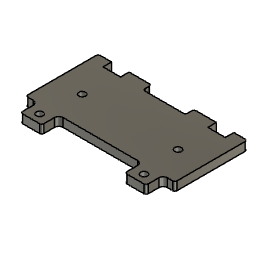
headcamera_plate_1 (Autodesk Fusion 360 design; units mm, degrees)
Autodesk Fusion 360 part; units mm, degrees
note: some values were not read from the file. Set by a fixed rule: the direction of a hole.
sketch "スケッチ1" plane through (0, 0, 0) normal (0, 0, 1) x (1, 0, 0)
  line L0 (-20.5, 20) -> (20.5, 20)
  line L1 (20.5, 20) -> (20.5, 16)
  line L2 (20.5, 16) -> (28.7, 16)
  line L3 (28.7, 16) -> (28.7, 20)
  line L4 (28.7, 20) -> (35, 20)
  line L5 (35, 20) -> (35, -14)
  line L6 (35, -14) -> (29.5, -14)
  line L7 (29.5, -14) -> (29.5, -22)
  line L8 (29.5, -22) -> (19.5, -22)
  line L9 (19.5, -22) -> (19.5, -14)
  line L10 (19.5, -14) -> (-19.5, -14)
  line L11 (-19.5, -14) -> (-19.5, -22)
  line L12 (-19.5, -22) -> (-29.5, -22)
  line L13 (-29.5, -22) -> (-29.5, -14)
  line L14 (-29.5, -14) -> (-35, -14)
  line L15 (-35, -14) -> (-35, 20)
  line L16 (-35, 20) -> (-28.7, 20)
  line L17 (-28.7, 20) -> (-28.7, 16)
  line L18 (-28.7, 16) -> (-20.5, 16)
  line L19 (-20.5, 16) -> (-20.5, 20)
  line L20 (-22.5, 0) -> (22.5, 0)
  line L21 (-24.5, -22) -> (-24.5, -18)
  line L22 (24.5, -22) -> (24.5, -18)
  line L23 (-10, 16) -> (10, 16)
  line L24 (10, 16) -> (10, 20)
  line L25 (10, 20) -> (-10, 20)
  line L26 (-10, 20) -> (-10, 16)
  point P0 (0, 20)
  point P1 (0, -14)
  dimension "d1" = 16
  dimension "d2" = 4
  dimension "d4" = 14
  dimension "d5" = 8
  dimension "d6" = 41
  dimension "d7" = 8.2
  dimension "d8" = 8.2
  dimension "d9" = 70
  dimension "d10" = 45
  dimension "d16" = 39
  dimension "d17" = 10
  dimension "d18" = 10
  dimension "d19" = 4
  dimension "d24" = 20
  dimension "d25" = 4
  constraint horizontal L0
  constraint perpendicular L0 L1
  constraint perpendicular L1 L2
  constraint perpendicular L2 L3
  constraint perpendicular L3 L4
  constraint perpendicular L4 L5
  constraint perpendicular L5 L6
  constraint perpendicular L4 L7
  constraint perpendicular L5 L8
  constraint perpendicular L8 L9
  constraint perpendicular L9 L10
  constraint perpendicular L8 L11
  constraint perpendicular L11 L12
  constraint perpendicular L8 L13
  constraint perpendicular L13 L14
  constraint perpendicular L14 L15
  constraint perpendicular L15 L16
  constraint perpendicular L16 L17
  constraint perpendicular L15 L18
  constraint perpendicular L0 L19
  constraint coincident L0.start L19.end
  constraint midpoint L0 P0
  constraint midpoint L10 P1
  constraint vertical origin P1
  constraint vertical origin P0
  constraint collinear L2 L18
  constraint collinear L0 L16
  constraint collinear L0 L4
  constraint collinear L6 L10
  constraint collinear L10 L14
  constraint collinear L8 L12
  constraint equal L4 L16
  constraint horizontal L20
  constraint midpoint origin L20
  constraint midpoint L12 L21.start
  constraint perpendicular L12 L21
  constraint midpoint L8 L22.start
  constraint perpendicular L8 L22
  constraint equal L21 L22
  constraint horizontal L23
  constraint vertical L24
  constraint horizontal L25
  constraint vertical L26
  constraint midpoint P0 L25
  measures "d1" distance of origin L2
  measures "d2" distance of L2.end L3.end
  measures "d4" distance of origin L6
  measures "d5" distance of L6 L8
  measures "d6" distance of L0.start L0.end
  measures "d7" distance of L1.end L2.end
  measures "d8" distance of L17.end L18.end
  measures "d9" distance of L5 L15
  measures "d10" distance of L20.start L20.end
  measures "d16" distance of L9.end L10.end
  measures "d17" distance of L11.end L12.end
  measures "d18" distance of L7 L9
  measures "d19" distance of L21.start L21.end
  measures "d24" distance of L24 L26
  measures "d25" distance of L23.end L24.end
extrude "押し出し1" add sketch "スケッチ1" along normal blind 4 contours L0 L1 L2 L3 L4 L5 L6 L7 L8 L9 L10 L11 L12 L13 L14 L15 L16 L17 L18 L19 L23 L24 L26
hole "穴1" at (-22.5, 0, 0) at (22.5, 0, 0) at (-24.5, -18, 0) at (24.5, -18, 0) direction (0, 0, 1) diameter 3.2 end through all
fillet "フィレット1" radius 1 12 edges at (35, 20, 2) (35, -14, 2) (29.5, -22, 2) (19.5, -22, 2) (-19.5, -22, 2) (-29.5, -22, 2) (-35, -14, 2) (-35, 20, 2) (10, 20, 2) (-10, 20, 2) (10, 16, 2) (-10, 16, 2)
fillet "フィレット2" radius 2 4 edges at (29.5, -14, 2) (19.5, -14, 2) (-19.5, -14, 2) (-29.5, -14, 2)
